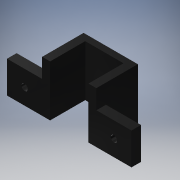
# Autodesk Inventor part: learnbotEncajeMotor
Saved by Autodesk Inventor 2017 (Build 210142000, 142)
## iProperties
Part Number: learnbotEncajeMotor
Material: Genérico
Document SubType Name: Modeling
Designer: rober
Density: 1 g/cm^3
Appearance: Valor por defecto
Author: rober
Autodesk Inventor part; units mm, degrees
ref_plane "YZ Plane" through (0, 0, 0) normal (1, 0, 0) x (0, 1, 0)
ref_plane "XZ Plane" through (0, 0, 0) normal (0, 1, 0) x (-1, 0, 0)
ref_plane "XY Plane" through (0, 0, 0) normal (0, 0, 1) x (1, 0, 0)
sketch "Boceto1" plane through (0, 0, 0) normal (0, 0, 1) x (1, 0, 0)
  line L0 (2.8, 1.3) -> (2.8, 0.3)
  line L1 (2.6, 0) -> (3.9, 0)
  line L2 (3.9, 0) -> (3.9, 0.3)
  line L3 (3.9, 0.3) -> (2.8, 0.3)
  line L4 (0, 0) -> (0, 0.3)
  line L5 (0, 0.3) -> (1.1, 0.3)
  line L6 (0, 0) -> (1.3, 0)
  line L7 (1.1, 1.3) -> (1.1, 0.3)
  line L8 (1.1, 1.3) -> (2.8, 1.3)
  line L9 (1.35, 1.1) -> (2.55, 1.1)
  line L10 (1.3, 0) -> (1.35, 0)
  line L11 (2.6, 0) -> (2.55, 0)
  line L12 (2.55, 0) -> (2.55, 1.1)
  line L13 (1.35, 0) -> (1.35, 1.1)
  dimension "d0" = 1
  dimension "d10" = 0.05
  dimension "d11" = 0.05
  constraints: 28 end point, 2 perpendicular, 1 horizontal
  measures "d10" distance of L6.end L10.end
  measures "d11" distance of L1.start L11.end
extrude "Extrusión1" add sketch "Boceto1" against normal blind 1
sketch "Boceto2" plane through (0, 0, 0) normal (0, 0, 1) x (1, 0, 0)
  line L0 (1.1, 0.3) -> (1.1, 1.3)
  line L1 (1.1, 1.3) -> (2.8, 1.3) projected
  line L2 (1.1, 1.3) -> (2.8, 1.3)
  line L3 (2.8, 1.3) -> (2.8, 0.3) projected
  line L4 (2.8, 1.3) -> (2.8, 0.3)
  line L5 (2.55, 0) -> (2.55, 1.1) projected
  line L6 (1.35, 1.1) -> (2.55, 1.1)
  line L7 (2.55, 1.1) -> (2.55, 0)
  line L8 (2.55, 0) -> (2.8, 0)
  line L9 (1.35, 1.1) -> (1.35, 0)
  line L10 (1.35, 0) -> (1.1, 0)
  line L11 (1.1, 0.3) -> (1.1, 1.3) projected
  line L12 (1.1, 0.3) -> (1.1, 0)
  line L13 (2.8, 0.3) -> (2.8, 0)
  constraints: 20 end point, 4 vertical, 3 perpendicular, 2 collinear, 1 horizontal
extrude "Extrusión2" add sketch "Boceto2" along normal blind 0.6
sketch "Boceto3" plane through (2.8, 0.3, 0) normal (0, 1, 0) x (1, 0, 0)
  line L0 (-1.7, 0) -> (-1.7, 1.9)
  line L1 (-1.7, 1.9) -> (0, 1.9)
  line L2 (0, 1.9) -> (0, 0)
  line L3 (0, 0) -> (-1.7, 0)
  line L4 (-1.7, 0) -> (-2.8, 0)
  line L5 (-2.8, 0) -> (-2.8, 1)
  line L6 (-2.8, 1) -> (-1.7, 1)
  line L7 (0, 0) -> (1.1, 0)
  line L8 (1.1, 0) -> (1.1, 1)
  line L9 (1.1, 1) -> (0, 1)
  circle A0 centre (-2.25, 0.5) radius 0.1
  circle A1 centre (0.55, 0.5) radius 0.1
  line L10 (1.1, 0) -> (0, 0) projected
  line L11 (1.1, 0) -> (1.1, 1) projected
  line L12 (0, 1) -> (1.1, 1) projected
  line L13 (0, 0) -> (0, 1) projected
  point P0 (-2.8, 0)
  dimension "d0" = 1
  dimension "d7" = 0.2
  dimension "d8" = 0.2
  constraints: 20 end point, 2 centre point, 2 point on line
  measures "d7" diameter of A1
  measures "d8" diameter of A0
extrude "Extrusión3" cut sketch "Boceto3" against normal blind 0.9 contours A0 | A1
